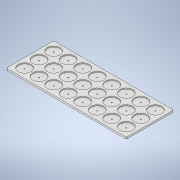
# Autodesk Inventor part: CC-topPlate
Saved by Autodesk Inventor 2020 (Build 240168000, 168)
## iProperties
Created: 2019-05-04
Part Number: CC-topPlate
Material: Acetal Resin, White
Document SubType Name: Modeling
Designer: andwh
Density: 1.425 g/cm^3
Appearance: Smooth - White
Author: andwh
Autodesk Inventor part; units mm, degrees
ref_plane "YZ Plane" through (0, 0, 0) normal (1, 0, 0) x (0, 1, 0)
ref_plane "XZ Plane" through (0, 0, 0) normal (0, 1, 0) x (-1, 0, 0)
ref_plane "XY Plane" through (0, 0, 0) normal (0, 0, 1) x (1, 0, 0)
sketch "Sketch1" plane through (0, 0, 0) normal (0, 1, 0) x (-1, 0, 0)
  line L0 (0, 0) -> (-838.2, 0)
  line L1 (-838.2, 0) -> (-838.2, -330.2)
  line L2 (-838.2, -330.2) -> (0, -330.2)
  line L3 (0, -330.2) -> (0, 0)
  circle A0 centre (-63.5, -63.5) radius 44.45
  circle A1 centre (-63.5, -165.1) radius 44.45
  circle A2 centre (-63.5, -266.7) radius 44.45
  circle A3 centre (-165.1, -63.5) radius 44.45
  circle A4 centre (-165.1, -165.1) radius 44.45
  circle A5 centre (-165.1, -266.7) radius 44.45
  circle A6 centre (-266.7, -63.5) radius 44.45
  circle A7 centre (-266.7, -165.1) radius 44.45
  circle A8 centre (-266.7, -266.7) radius 44.45
  circle A9 centre (-368.3, -63.5) radius 44.45
  circle A10 centre (-368.3, -165.1) radius 44.45
  circle A11 centre (-368.3, -266.7) radius 44.45
  circle A12 centre (-469.9, -63.5) radius 44.45
  circle A13 centre (-469.9, -165.1) radius 44.45
  circle A14 centre (-469.9, -266.7) radius 44.45
  circle A15 centre (-571.5, -63.5) radius 44.45
  circle A16 centre (-571.5, -165.1) radius 44.45
  circle A17 centre (-571.5, -266.7) radius 44.45
  circle A18 centre (-673.1, -63.5) radius 44.45
  circle A19 centre (-673.1, -165.1) radius 44.45
  circle A20 centre (-673.1, -266.7) radius 44.45
  circle A21 centre (-774.7, -63.5) radius 44.45
  circle A22 centre (-774.7, -165.1) radius 44.45
  circle A23 centre (-774.7, -266.7) radius 44.45
  circle A24 centre (-25.4, -76.2) radius 2.0193
  circle A25 centre (-101.6, -76.2) radius 2.0193
  circle A26 centre (-25.4, -50.8) radius 2.0193
  circle A27 centre (-101.6, -50.8) radius 2.0193
  line L4 (-63.5, -68.5) -> (-63.5, -39.5) construction
  line L5 (-46, -68.5) -> (-46, -39.5) construction
  line L6 (-81, -39.5) -> (-81, -68.5) construction
  arc A28 (-81, -68.5) -> (-46, -68.5) centre (-63.5, -68.5) ccw construction
  arc A29 (-46, -39.5) -> (-81, -39.5) centre (-63.5, -39.5) ccw construction
  circle A30 centre (-63.5, -63.5) radius 3.5
  circle A31 centre (-51.5, -54) radius 1.775 construction
  line L7 (-72.5, -79) -> (-72.5, -29) construction
  circle A32 centre (-72.5, -79) radius 1.775 construction
  circle A33 centre (-72.5, -29) radius 1.775 construction
  line L8 (-52.07, -73.38) -> (-74.93, -73.38) construction
  line L9 (-52.07, -65.62) -> (-52.07, -42.38) construction
  circle A34 centre (-52.07, -73.38) radius 0.65 construction
  circle A35 centre (-52.07, -65.62) radius 0.65 construction
  circle A36 centre (-52.07, -42.38) radius 0.65 construction
  circle A37 centre (-52.07, -34.62) radius 0.65 construction
  circle A38 centre (-74.93, -34.62) radius 0.65 construction
  circle A39 centre (-74.93, -42.38) radius 0.65 construction
  circle A40 centre (-74.93, -65.62) radius 0.65 construction
  circle A41 centre (-74.93, -73.38) radius 0.65 construction
  circle A42 centre (-127, -50.8) radius 2.0193
  circle A43 centre (-127, -76.2) radius 2.0193
  circle A44 centre (-165.1, -63.5) radius 3.5
  circle A45 centre (-203.2, -76.2) radius 2.0193
  circle A46 centre (-203.2, -50.8) radius 2.0193
  circle A47 centre (-228.6, -50.8) radius 2.0193
  circle A48 centre (-228.6, -76.2) radius 2.0193
  circle A49 centre (-266.7, -63.5) radius 3.5
  circle A50 centre (-304.8, -76.2) radius 2.0193
  circle A51 centre (-304.8, -50.8) radius 2.0193
  circle A52 centre (-330.2, -50.8) radius 2.0193
  circle A53 centre (-330.2, -76.2) radius 2.0193
  circle A54 centre (-368.3, -63.5) radius 3.5
  circle A55 centre (-406.4, -76.2) radius 2.0193
  circle A56 centre (-406.4, -50.8) radius 2.0193
  circle A57 centre (-431.8, -50.8) radius 2.0193
  circle A58 centre (-431.8, -76.2) radius 2.0193
  circle A59 centre (-469.9, -63.5) radius 3.5
  circle A60 centre (-508, -76.2) radius 2.0193
  circle A61 centre (-508, -50.8) radius 2.0193
  circle A62 centre (-533.4, -50.8) radius 2.0193
  circle A63 centre (-533.4, -76.2) radius 2.0193
  circle A64 centre (-571.5, -63.5) radius 3.5
  circle A65 centre (-609.6, -76.2) radius 2.0193
  circle A66 centre (-609.6, -50.8) radius 2.0193
  circle A67 centre (-635, -50.8) radius 2.0193
  circle A68 centre (-635, -76.2) radius 2.0193
  circle A69 centre (-673.1, -63.5) radius 3.5
  circle A70 centre (-711.2, -76.2) radius 2.0193
  circle A71 centre (-711.2, -50.8) radius 2.0193
  circle A72 centre (-736.6, -50.8) radius 2.0193
  circle A73 centre (-736.6, -76.2) radius 2.0193
  circle A74 centre (-774.7, -63.5) radius 3.5
  circle A75 centre (-812.8, -76.2) radius 2.0193
  circle A76 centre (-812.8, -50.8) radius 2.0193
  circle A77 centre (-25.4, -152.4) radius 2.0193
  circle A78 centre (-25.4, -177.8) radius 2.0193
  circle A79 centre (-63.5, -165.1) radius 3.5
  circle A80 centre (-101.6, -177.8) radius 2.0193
  circle A81 centre (-101.6, -152.4) radius 2.0193
  circle A82 centre (-127, -152.4) radius 2.0193
  circle A83 centre (-127, -177.8) radius 2.0193
  circle A84 centre (-165.1, -165.1) radius 3.5
  circle A85 centre (-203.2, -177.8) radius 2.0193
  circle A86 centre (-203.2, -152.4) radius 2.0193
  circle A87 centre (-228.6, -152.4) radius 2.0193
  circle A88 centre (-228.6, -177.8) radius 2.0193
  circle A89 centre (-266.7, -165.1) radius 3.5
  circle A90 centre (-304.8, -177.8) radius 2.0193
  circle A91 centre (-304.8, -152.4) radius 2.0193
  circle A92 centre (-330.2, -152.4) radius 2.0193
  circle A93 centre (-330.2, -177.8) radius 2.0193
  circle A94 centre (-368.3, -165.1) radius 3.5
  circle A95 centre (-406.4, -177.8) radius 2.0193
  circle A96 centre (-406.4, -152.4) radius 2.0193
  circle A97 centre (-431.8, -152.4) radius 2.0193
  circle A98 centre (-431.8, -177.8) radius 2.0193
  circle A99 centre (-469.9, -165.1) radius 3.5
  circle A100 centre (-508, -177.8) radius 2.0193
  circle A101 centre (-508, -152.4) radius 2.0193
  circle A102 centre (-533.4, -152.4) radius 2.0193
  circle A103 centre (-533.4, -177.8) radius 2.0193
  circle A104 centre (-571.5, -165.1) radius 3.5
  circle A105 centre (-609.6, -177.8) radius 2.0193
  circle A106 centre (-609.6, -152.4) radius 2.0193
  circle A107 centre (-635, -152.4) radius 2.0193
  circle A108 centre (-635, -177.8) radius 2.0193
  circle A109 centre (-673.1, -165.1) radius 3.5
  circle A110 centre (-711.2, -177.8) radius 2.0193
  circle A111 centre (-711.2, -152.4) radius 2.0193
  circle A112 centre (-736.6, -152.4) radius 2.0193
  circle A113 centre (-736.6, -177.8) radius 2.0193
  circle A114 centre (-774.7, -165.1) radius 3.5
  circle A115 centre (-812.8, -177.8) radius 2.0193
  circle A116 centre (-812.8, -152.4) radius 2.0193
  circle A117 centre (-25.4, -254) radius 2.0193
  circle A118 centre (-25.4, -279.4) radius 2.0193
  circle A119 centre (-63.5, -266.7) radius 3.5
  circle A120 centre (-101.6, -279.4) radius 2.0193
  circle A121 centre (-101.6, -254) radius 2.0193
  circle A122 centre (-127, -254) radius 2.0193
  circle A123 centre (-127, -279.4) radius 2.0193
  circle A124 centre (-165.1, -266.7) radius 3.5
  circle A125 centre (-203.2, -279.4) radius 2.0193
  circle A126 centre (-203.2, -254) radius 2.0193
  circle A127 centre (-228.6, -254) radius 2.0193
  circle A128 centre (-228.6, -279.4) radius 2.0193
  circle A129 centre (-266.7, -266.7) radius 3.5
  circle A130 centre (-304.8, -279.4) radius 2.0193
  circle A131 centre (-304.8, -254) radius 2.0193
  circle A132 centre (-330.2, -254) radius 2.0193
  circle A133 centre (-330.2, -279.4) radius 2.0193
  circle A134 centre (-368.3, -266.7) radius 3.5
  circle A135 centre (-406.4, -279.4) radius 2.0193
  circle A136 centre (-406.4, -254) radius 2.0193
  circle A137 centre (-431.8, -254) radius 2.0193
  circle A138 centre (-431.8, -279.4) radius 2.0193
  circle A139 centre (-469.9, -266.7) radius 3.5
  circle A140 centre (-508, -279.4) radius 2.0193
  circle A141 centre (-508, -254) radius 2.0193
  circle A142 centre (-533.4, -254) radius 2.0193
  circle A143 centre (-533.4, -279.4) radius 2.0193
  circle A144 centre (-571.5, -266.7) radius 3.5
  circle A145 centre (-609.6, -279.4) radius 2.0193
  circle A146 centre (-609.6, -254) radius 2.0193
  circle A147 centre (-635, -254) radius 2.0193
  circle A148 centre (-635, -279.4) radius 2.0193
  circle A149 centre (-673.1, -266.7) radius 3.5
  circle A150 centre (-711.2, -279.4) radius 2.0193
  circle A151 centre (-711.2, -254) radius 2.0193
  circle A152 centre (-736.6, -254) radius 2.0193
  circle A153 centre (-736.6, -279.4) radius 2.0193
  circle A154 centre (-774.7, -266.7) radius 3.5
  circle A155 centre (-812.8, -279.4) radius 2.0193
  circle A156 centre (-812.8, -254) radius 2.0193
  point P0 (-63.5, -54)
  point P1 (-63.5, -86)
  point P2 (-63.5, -22)
  point P3 (-72.5, -54)
  point P4 (-63.5, -73.38)
  point P5 (-52.07, -54)
  dimension "d2" = 88.9
  dimension "d3" = 63.5
  dimension "d4" = 63.5
  dimension "d7" = 101.6
  dimension "d10" = 101.6
  dimension "d13" = 63.5
  dimension "d14" = 63.5
  dimension "d15" = 838.2
  dimension "d16" = 330.2
  dimension "d44" = 4.0386
  dimension "d49" = 76.2
  dimension "d52" = 25.4
  dimension "d72" = 17.5
  dimension "d73" = 9.5
  dimension "d74" = 7
  dimension "d75" = 64
  dimension "d76" = 3.55
  dimension "d77" = 12
  dimension "d78" = 50
  dimension "d79" = 9
  dimension "d80" = 22.86
  dimension "d81" = 7.76
  dimension "d82" = 7.76
  dimension "d83" = 23.24
  dimension "d84" = 1.3
  dimension "d126" = 12.7
  dimension "d127" = 38.1
  dimension "d130" = 101.6
  dimension "d133" = 101.6
  constraints: 157 centre point, 22 end point, 11 coincident, 9 equal radius, 7 vertical alignment, 6 horizontal alignment, 6 point on circle, 6 vertical, 5 horizontal, 4 midpoint, 4 tangent, 3 parallel, 1 perpendicular, 1 point on line, 282 other
  measures "d2" diameter of A0
  measures "d3" distance from line of L3 A0.centre
  measures "d4" distance from line of L0 A0.centre
  measures "d7" distance of A0.centre A1.centre
  measures "d10" distance of A0.centre A3.centre
  measures "d13" distance from line of A2.centre L2
  measures "d14" distance from line of A21.centre L1
  measures "d15" distance of L1.end L2.end
  measures "d16" distance of L0.end L1.end
  measures "d44" diameter of A24
  measures "d49" distance of A24.centre A25.centre
  measures "d52" distance of A24.centre A26.centre
  measures "d72" radius of A28
  measures "d73" distance of point (-63.5, -54) A30.centre
  measures "d74" diameter of A30
  measures "d75" distance of point (-63.5, -22) point (-63.5, -86)
  measures "d76" diameter of A31
  measures "d77" distance from line of L4 A31.centre
  measures "d78" distance of L7.start L7.end
  measures "d79" distance between parallel lines of L4 L7
  measures "d80" distance of L8.start L8.end
  measures "d81" distance of L9.start L8.start
  measures "d82" distance of point (-52.07, -34.62) L9.end
  measures "d83" distance of L9.start L9.end
  measures "d84" diameter of A34
  measures "d126" vertical distance of A0.centre A24.centre
  measures "d127" horizontal distance of A24.centre A0.centre
  measures "d130" distance of A26.centre A42.centre
  measures "d133" distance of A26.centre A77.centre
extrude "Extrusion1" add sketch "Sketch1" against normal blind 4.7625 contours L3 L2 L1 L0 | A0 | A1 | A2 | A3 | A4 | A5 | A6 | A7 | A8 | A9 | A10 | A11 | A12 | A13 | A14 | A15 | A16 | A17 | A18 | A19 | A20 | A21 | A22 | A23
sketch "Sketch2" plane through (0, 0, 0) normal (0, 1, 0) x (1, 0, 0)
  line L0 (0, 0) -> (838.2, 0) projected
  line L1 (838.2, 0) -> (838.2, 330.2) projected
  line L2 (838.2, 330.2) -> (0, 330.2) projected
  line L3 (0, 330.2) -> (0, 0) projected
  circle A0 centre (63.5, 266.7) radius 3.5 projected
  circle A1 centre (63.5, 165.1) radius 3.5 projected
  circle A2 centre (63.5, 63.5) radius 3.5 projected
  circle A3 centre (165.1, 63.5) radius 3.5 projected
  circle A4 centre (165.1, 165.1) radius 3.5 projected
  circle A5 centre (165.1, 266.7) radius 3.5 projected
  circle A6 centre (266.7, 266.7) radius 3.5 projected
  circle A7 centre (368.3, 266.7) radius 3.5 projected
  circle A8 centre (469.9, 266.7) radius 3.5 projected
  circle A9 centre (571.5, 266.7) radius 3.5 projected
  circle A10 centre (673.1, 266.7) radius 3.5 projected
  circle A11 centre (774.7, 266.7) radius 3.5 projected
  circle A12 centre (774.7, 165.1) radius 3.5 projected
  circle A13 centre (774.7, 63.5) radius 3.5 projected
  circle A14 centre (673.1, 63.5) radius 3.5 projected
  circle A15 centre (673.1, 165.1) radius 3.5 projected
  circle A16 centre (571.5, 165.1) radius 3.5 projected
  circle A17 centre (571.5, 63.5) radius 3.5 projected
  circle A18 centre (469.9, 63.5) radius 3.5 projected
  circle A19 centre (469.9, 165.1) radius 3.5 projected
  circle A20 centre (368.3, 165.1) radius 3.5 projected
  circle A21 centre (368.3, 63.5) radius 3.5 projected
  circle A22 centre (266.7, 63.5) radius 3.5 projected
  circle A23 centre (266.7, 165.1) radius 3.5 projected
extrude "Extrusion2" add sketch "Sketch2" along normal blind 1.5875
sketch "Sketch3" plane through (0, 1.5875, 0) normal (0, 1, 0) x (1, 0, 0)
  line L0 (0, 330.2) -> (0, 0) projected
  line L1 (838.2, 330.2) -> (0, 330.2) projected
  line L2 (838.2, 0) -> (838.2, 330.2) projected
  line L3 (0, 0) -> (838.2, 0) projected
  circle A0 centre (63.5, 63.5) radius 3.5 projected
  circle A1 centre (63.5, 63.5) radius 44.45
  circle A2 centre (63.5, 165.1) radius 44.45
  circle A3 centre (63.5, 266.7) radius 44.45
  circle A4 centre (165.1, 63.5) radius 44.45
  circle A5 centre (165.1, 165.1) radius 44.45
  circle A6 centre (165.1, 266.7) radius 44.45
  circle A7 centre (266.7, 63.5) radius 44.45
  circle A8 centre (266.7, 165.1) radius 44.45
  circle A9 centre (266.7, 266.7) radius 44.45
  circle A10 centre (368.3, 63.5) radius 44.45
  circle A11 centre (368.3, 165.1) radius 44.45
  circle A12 centre (368.3, 266.7) radius 44.45
  circle A13 centre (469.9, 63.5) radius 44.45
  circle A14 centre (469.9, 165.1) radius 44.45
  circle A15 centre (469.9, 266.7) radius 44.45
  circle A16 centre (571.5, 63.5) radius 44.45
  circle A17 centre (571.5, 165.1) radius 44.45
  circle A18 centre (571.5, 266.7) radius 44.45
  circle A19 centre (673.1, 63.5) radius 44.45
  circle A20 centre (673.1, 165.1) radius 44.45
  circle A21 centre (673.1, 266.7) radius 44.45
  circle A22 centre (774.7, 63.5) radius 44.45
  circle A23 centre (774.7, 165.1) radius 44.45
  circle A24 centre (774.7, 266.7) radius 44.45
  dimension "d140" = 88.9
  dimension "d143" = 101.6
  dimension "d146" = 101.6
  constraints: 24 centre point, 1 coincident, 1 horizontal, 1 vertical, 46 other
  measures "d140" diameter of A1
  measures "d143" distance of A1.centre A2.centre
  measures "d146" distance of A1.centre A4.centre
extrude "Extrusion3" add sketch "Sketch3" along normal blind 6.35 contours L1 L2 L3 L0
fillet "Fillet1" radius 6.35 4 edges at (0, 1.5875, 0) (838.2, 1.5875, 0) (838.2, 1.5875, -330.2) (0, 1.5875, -330.2)
equation "\"d13\" = d4"
equation "\"d14\" = d3"
body "Solid1"
